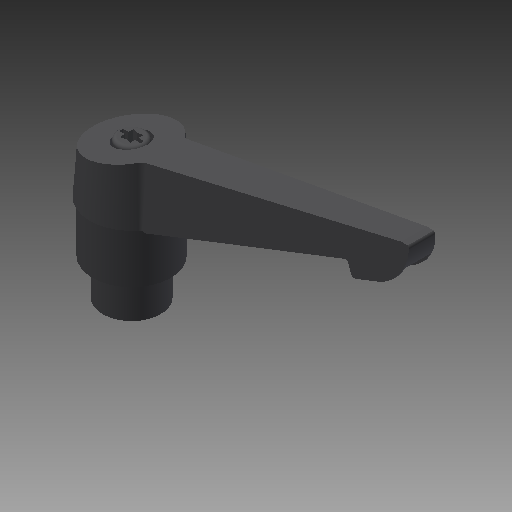
# Autodesk Inventor part: May Tec 1.63.14041_Clamping lever 80
Saved by Autodesk Inventor 2018 (Build 220112000, 112)
## iProperties
Category: PARTsolutions
Company: MAYTEC
Created: 2012-12-11
Part Number: May Tec 1.63.14041_Clamping lever 80
Catalog Web Link: www.cadenas.de
Description: 1.29.x-Lever
Vendor: MAYTEC
Document SubType Name: Modeling
Designer: PARTuser1
Manufacturer: MAYTEC
Density: 1 g/cm^3
Material: Generic
Appearance: RGB(0.00000000000000,0.00000000000000,0.00000000000000)
PSOL_IDENT_0: {\\10.0.0.242\data_v9\23d-libs\maytec\maytec_3d\anbauzubehoer\gelenke\gelenke_pg_30-50_spannhebel\he
PSOL_IDENT_1: bel_pg_20-30.prj},215 {VTYP=3D},{NB=May Tec 1.63.14041_Clamping lever 80},{LINA=May Tec 1.63.14041_C
PSOL_IDENT_2: lamping lever 80},{NN=1.29.x},{DATE=14.09.2010 08:31:39},{GEOMDATE=15.02.2008 00:00:00},{VERSION=},{
PSOL_IDENT_3: LINEID=140},{LINESUBID=-1},{WBVAR=}  {NB=May Tec 1.63.14041_Clamping lever 80},{LINA=May Tec 1.63.14
PSOL_IDENT_4: 041_Clamping lever 80},{KT=DUMMY},{IDNR=},{PARTNR=1.63.14041},{DESCRIPTION=Spannhebel 80},{M1=10.0},
PSOL_IDENT_5: {T=14.0},{A=80.0},{A1=92.0},{B=11.0},{D=16.0},{D1=21.5},{D2=23.0},{H=37.5},{H1=10.0},{H2=24.0},{H3=5
PSOL_IDENT_6: 3.0},{H4=57.0},{XTRANS=Clamping lever 80}
CNS_NT: Lever
CNS_NB: May Tec 1.63.14041_Clamping lever 80
CNS_NBSYN: May Tec $PARTNR._$XTRANS.
CNS_LINA: May Tec 1.63.14041_Clamping lever 80
CNS_PARTNR: 1.63.14041
CNS_DESCRIPTION: Clamping lever 80
CNS_M1: 10.0
CNS_T: 14.0
CNS_A: 80.0
CNS_A1: 92.0
CNS_B: 11.0
CNS_D: 16.0
CNS_D1: 21.5
CNS_D2: 23.0
CNS_H: 37.5
CNS_H1: 10.0
CNS_H2: 24.0
CNS_H3: 53.0
CNS_H4: 57.0
CNS_XTRANS: Clamping lever 80
SUPPLIER: MAYTEC
ARTICLENO: May Tec 1.63.14041_Clamping lever 80
BOMINFO: May Tec 1.63.14041_Clamping lever 80
CREATOR: CADENAS GmbH
Title: May Tec 1.63.14041_Clamping lever 80
Author: Cadenas PARTsolutions
Comments: Lever
Autodesk Inventor part; units mm, degrees
sketch "Skizze_1" plane through (0, 0, 0) normal (0, 0, 1) x (1, 0, 0)
  line L0 (0, 10) -> (0, 24)
  line L1 (0, 24) -> (10.75, 24)
  line L2 (10.75, 24) -> (10.75, 10)
  line L3 (10.75, 10) -> (0, 10)
  line L4 (0, 10) -> (0, 24)
  constraints: 10 end point
revolve "Revolution1" add sketch "Skizze_1" angle 360 about axis through (0, 10, 0) along (0, -1, 0)
sketch "Skizze_2" plane through (0, 0, 0) normal (0, 0, 1) x (1, 0, 0)
  line L0 (0, 37.5) -> (0, 24)
  line L1 (0, 24) -> (-10.9041, 24)
  arc A0 (-11.3965, 24.5868) -> (-10.9041, 24) centre (-10.9041, 24.5) ccw
  line L2 (-11.3965, 24.5868) -> (-10.3942, 30.2711)
  arc A1 (-6.7643, 34.2325) -> (-10.3942, 30.2711) centre (-5.4702, 29.4029) ccw
  line L3 (-6.7643, 34.2325) -> (-3.9, 35)
  line L4 (-3.9, 35) -> (-3.9, 37.5)
  line L5 (-3.9, 37.5) -> (0, 37.5)
  line L6 (0, 37.5) -> (0, 24)
  constraints: 14 end point, 4 point on circle, 2 centre point
revolve "Revolution2" add sketch "Skizze_2" angle 360 about axis through (0, 37.5, 0) along (0, 1, 0)
sketch "Skizze_4" plane through (0, 24, 0) normal (0, 1, 0) x (1, 0, 0)
  arc A0 (9.0089, 7.1477) -> (9.0089, -7.1477) centre (0, 0) ccw
  arc A1 (9.7748, -6.7694) -> (9.0089, -7.1477) centre (9.7923, -7.7693) ccw
  line L0 (9.7748, -6.7694) -> (80.5349, -5.5343)
  arc A2 (80.5349, -5.5343) -> (82.5, -3.5346) centre (80.5, -3.5346) ccw
  line L1 (82.5, -3.5346) -> (82.5, 3.5346)
  arc A3 (82.5, 3.5346) -> (80.5349, 5.5343) centre (80.5, 3.5346) ccw
  line L2 (80.5349, 5.5343) -> (9.7748, 6.7694)
  arc A4 (9.0089, 7.1477) -> (9.7748, 6.7694) centre (9.7923, 7.7693) ccw
  constraints: 10 point on circle, 6 end point, 5 centre point
extrude "Extrusion1" add sketch "Skizze_4" along normal blind 30 draft -3.8
sketch "Skizze_3" plane through (0, 0, 0) normal (0, 0, 1) x (1, 0, 0)
  line L0 (-12.75, 35.0297) -> (78.7943, 54.201)
  arc A0 (79.9992, 53.2105) -> (78.7943, 54.201) centre (78.9992, 53.2222) ccw
  arc A1 (72.1042, 42.0744) -> (79.9992, 53.2105) centre (68, 53.3507) ccw
  line L1 (72.1042, 42.0744) -> (66.333, 39.9738)
  arc A2 (65.0513, 40.5715) -> (66.333, 39.9738) centre (65.991, 40.9135) ccw
  line L2 (65.0513, 40.5715) -> (64.3672, 42.4509)
  arc A3 (64.3672, 42.4509) -> (63.0855, 43.0486) centre (63.4276, 42.1089) ccw
  line L3 (63.0855, 43.0486) -> (10.75, 24)
  line L4 (10.75, 24) -> (10.75, 0)
  line L5 (10.75, 0) -> (83, 0)
  line L6 (83, 0) -> (83, 73)
  line L7 (83, 73) -> (-12.75, 73)
  line L8 (-12.75, 73) -> (-12.75, 35.0297)
  constraints: 18 end point, 8 point on circle, 4 centre point
extrude "Extrusion2" cut sketch "Skizze_3" along normal mid plane 50
sketch "Skizze_5" plane through (0, 24, 0) normal (0, 1, 0) x (1, 0, 0)
  circle A0 centre (0, 0) radius 4.325
  constraints: 1 centre point
extrude "Extrusion3" cut sketch "Skizze_5" along normal blind 25
sketch "Skizze_6" plane through (0, 0, 0) normal (0, 0, 1) x (1, 0, 0)
  line L0 (0, 24) -> (0, 38.5)
  line L1 (0, 38.5) -> (2.925, 38.5)
  arc A0 (3.925, 37.5) -> (2.925, 38.5) centre (2.925, 37.5) ccw
  line L2 (3.925, 37.5) -> (3.925, 24)
  line L3 (3.925, 24) -> (0, 24)
  line L4 (0, 24) -> (0, 38.5)
  constraints: 10 end point, 2 point on circle, 1 centre point
revolve "Revolution3" add sketch "Skizze_6" angle 360 about axis through (0, 24, 0) along (0, -1, 0)
sketch "Skizze_7" plane through (0, 38.5, 0) normal (0, 1, 0) x (1, 0, 0)
  arc A0 (-2.8819, 0.5) -> (-2.8819, -0.5) centre (0, 0) ccw
  line L0 (-2.8819, -0.5) -> (-1.4, -0.5)
  line L1 (-1.4, -0.5) -> (-1.4, -1.875)
  line L2 (-1.4, -1.875) -> (0, -1.5)
  line L3 (0, -1.5) -> (1.4, -1.875)
  line L4 (1.4, -1.875) -> (1.4, -0.5)
  line L5 (1.4, -0.5) -> (2.8819, -0.5)
  arc A1 (2.8819, -0.5) -> (2.8819, 0.5) centre (0, 0) ccw
  line L6 (2.8819, 0.5) -> (1.4, 0.5)
  line L7 (1.4, 0.5) -> (1.4, 1.875)
  line L8 (1.4, 1.875) -> (0, 1.5)
  line L9 (0, 1.5) -> (-1.4, 1.875)
  line L10 (-1.4, 1.875) -> (-1.4, 0.5)
  line L11 (-1.4, 0.5) -> (-2.8819, 0.5)
  constraints: 24 end point, 4 point on circle, 2 centre point
extrude "Extrusion4" cut sketch "Skizze_7" against normal blind 3
sketch "Skizze_12" plane through (0, 0, 0) normal (0, 0, 1) x (1, 0, 0)
  line L0 (64.8831, 49.805) -> (68.4899, 39.8955)
  line L1 (68.4899, 39.8955) -> (80.2362, 44.1709)
  line L2 (80.2362, 44.1709) -> (77.6165, 51.3685)
  line L3 (77.6165, 51.3685) -> (64.8831, 49.805)
  constraints: 8 end point
extrude "Extrusion5" cut sketch "Skizze_12" along normal mid plane 7
sketch "Skizze_13" plane through (0, 0, 0) normal (0, 0, 1) x (1, 0, 0)
  line L0 (11.7761, 21.1809) -> (64.0792, 40.2177)
  line L1 (64.0792, 40.2177) -> (61.4289, 47.4992)
  line L2 (61.4289, 47.4992) -> (11.7761, 37.1009)
  line L3 (11.7761, 37.1009) -> (11.7761, 21.1809)
  constraints: 8 end point
extrude "Extrusion6" cut sketch "Skizze_13" along normal mid plane 6
sketch "Skizze_14" plane through (0, 0, 0) normal (0, 1, 0) x (-1, 0, 0)
  circle A0 centre (0, 0) radius 8
  constraints: 1 centre point
extrude "Extrusion7" add sketch "Skizze_14" along normal blind 10
sketch "Sketch11" plane through (0, 0, 0) normal (0, -1, 0) x (1, 0, 0)
  point P0 (0, 0)
hole "Drilling 2" at (0, 0, 0) direction (0, 1, 0) diameter 8.376 depth 14 countersink diameter 10 countersink angle 90 thread size "M10x1.5" class "6H" standard "ISO Metric profile"
ref_plane "fluegel_XY" through (0, 0, 0) normal (0, 1, 0) x (1, 0, 0)
ref_plane "fluegel_YZ" through (0, 0, 0) normal (1, 0, 0) x (0, 0, -1)
ref_plane "fluegel_ZX" through (0, 0, 0) normal (0, 0, -1) x (0, 1, 0)
body "Solid1"
